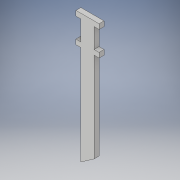
# Autodesk Inventor part: k2_t_leg
Saved by Autodesk Inventor 2017 (Build 210142000, 142)
## iProperties
Created: 2017-02-08
Part Number: k2_t_leg
Material: Generic
Document SubType Name: Modeling
Designer: herman
Density: 1 g/cm^3
Appearance: Default
Author: herman
Autodesk Inventor part; units mm, degrees
ref_plane "YZ Plane" through (0, 0, 0) normal (1, 0, 0) x (0, 1, 0)
ref_plane "XZ Plane" through (0, 0, 0) normal (0, 1, 0) x (-1, 0, 0)
ref_plane "XY Plane" through (0, 0, 0) normal (0, 0, 1) x (1, 0, 0)
sketch "Sketch2" plane through (0, 0, 0) normal (0, 0, 1) x (1, 0, 0)
  line L0 (-7.3607, 82.5814) -> (-7.3607, 22.5627)
  line L1 (-7.3607, 22.5627) -> (0.6393, 28.1644)
  line L2 (0.6393, 28.1644) -> (0.6393, 82.5814)
  line L3 (-7.3607, 82.5814) -> (-10.3607, 82.5814)
  line L4 (-10.3607, 82.5814) -> (-10.3607, 100.5814)
  line L5 (0.6393, 82.5814) -> (3.6393, 82.5814)
  line L6 (3.6393, 82.5814) -> (3.6393, 100.5814)
  line L7 (-10.3607, 100.5814) -> (3.6393, 100.5814)
  line L8 (-10.3607, 85.5814) -> (3.6393, 85.5814) construction
  point P0 (0, 0)
  dimension "d3" = 125
  dimension "d9" = 8
  dimension "d10" = 18
  dimension "d11" = 3
  dimension "d12" = 57.417
  dimension "d13" = 3
  dimension "d14" = 18
  constraints: 19 end point, 3 horizontal, 3 perpendicular, 2 point on line, 1 collinear, 1 parallel, 1 vertical
  measures "d3" angle of L2 L1
  measures "d9" distance of L2.end L0.start
  measures "d10" distance of L3.end L4.end
  measures "d11" distance between parallel lines of L8 L3
  measures "d12" distance from line of L1.end L8
  measures "d13" distance of L2.end L5.end
  measures "d14" distance of L5.end L6.end
extrude "Extrusion1" add sketch "Sketch2" along normal blind 3
sketch "Sketch3" plane through (0, 0, 3) normal (0, 0, 1) x (1, 0, 0)
  line L0 (-10.3607, 100.5814) -> (-10.3607, 82.5814) projected
  line L1 (3.6393, 82.5814) -> (3.6393, 100.5814) projected
  line L2 (-10.3607, 85.5814) -> (-7.3607, 85.5814)
  line L3 (-7.3607, 85.5814) -> (-7.3607, 97.5814)
  line L4 (-7.3607, 97.5814) -> (-10.3607, 97.5814)
  line L5 (-10.3607, 97.5814) -> (-10.3607, 85.5814)
  line L6 (3.6393, 85.5814) -> (0.6393, 85.5814)
  line L7 (0.6393, 85.5814) -> (0.6393, 97.5814)
  line L8 (0.6393, 97.5814) -> (3.6393, 97.5814)
  line L9 (3.6393, 97.5814) -> (3.6393, 85.5814)
  point P0 (0, 0)
  dimension "d15" = 3
  dimension "d16" = 12
  dimension "d17" = 3
  constraints: 16 end point, 4 parallel, 4 point on line, 2 horizontal, 2 perpendicular, 1 collinear
  measures "d15" distance of L3.end L4.end
  measures "d16" distance of L2.end L3.end
  measures "d17" distance of L0.end L2.start
extrude "Extrusion2" cut sketch "Sketch3" against normal through all
equation "\"d14\" = d10"
body "Solid2"
